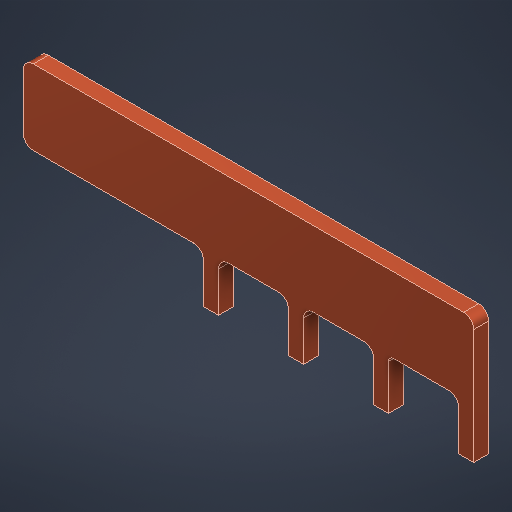
# Autodesk Inventor part: Bus_copper_GND
Saved by Autodesk Inventor 2026.2 (Build 302298000, 298)
## iProperties
Created: 2025-12-09
Part Number: Bus_copper_GND
Material: Медь
Document SubType Name: Modeling
Designer: EV-TECH
Density: 8.94 g/cm^3
Appearance: Медь — сатинированная
Author: EV-TECH
Autodesk Inventor part; units mm, degrees
ref_plane "YZ Plane" through (0, 0, 0) normal (1, 0, 0) x (0, 1, 0)
ref_plane "XZ Plane" through (0, 0, 0) normal (0, 1, 0) x (-1, 0, 0)
ref_plane "XY Plane" through (0, 0, 0) normal (0, 0, 1) x (1, 0, 0)
sketch "Эскиз1" plane through (0, 0, 0) normal (0, 1, 0) x (-1, 0, 0)
  line L0 (0, 0) -> (3, 0)
  line L1 (3, 0) -> (3, -3)
  line L2 (3, -3) -> (0, -3)
  line L3 (0, -3) -> (0, 0)
  line L4 (3, 0) -> (20, 0)
  line L5 (20, 0) -> (17, 0)
  line L6 (17, 0) -> (17, -3)
  line L7 (17, -3) -> (20, -3)
  line L8 (20, -3) -> (20, 0)
  line L9 (20, 0) -> (37, 0)
  line L10 (37, 0) -> (34, 0)
  line L11 (34, 0) -> (34, -3)
  line L12 (34, -3) -> (37, -3)
  line L13 (37, -3) -> (37, 0)
  line L14 (37, 0) -> (54, 0)
  line L15 (54, 0) -> (51, 0)
  line L16 (51, 0) -> (51, -3)
  line L17 (51, -3) -> (54, -3)
  line L18 (54, -3) -> (54, 0)
  point P0 (17, 0)
  point P1 (17, 0)
  dimension "d0" = 3
  dimension "d1" = 3
  dimension "d17" = 17
  dimension "d18" = 3
  dimension "d19" = 3
  dimension "d20" = 17
  dimension "d21" = 17
  dimension "d22" = 3
  dimension "d23" = 3
  dimension "d24" = 3
  dimension "d25" = 3
  constraints: 38 end point, 8 parallel, 7 horizontal, 4 perpendicular, 1 point on line
  measures "d0" distance of L1.end L2.end
  measures "d1" distance of L0.end L1.end
  measures "d17" distance of L0.end L4.end
  measures "d18" distance of L6.end L7.end
  measures "d19" distance of L7.end L4.end
  measures "d20" distance of L4.end L9.end
  measures "d21" distance of L9.end L14.end
  measures "d22" distance of L16.end L17.end
  measures "d23" distance of L17.end L14.end
  measures "d24" distance of L12.end L9.end
  measures "d25" distance of L11.end L12.end
extrude "Выдавливание1" add sketch "Эскиз1" along normal blind 10
sketch "Эскиз2" plane through (0, 10, 0) normal (0, 1, 0) x (1, 0, 0)
  line L0 (0, 0) -> (-90, 0)
  line L1 (-90, 0) -> (-90, 3)
  line L2 (-90, 3) -> (0, 3)
  line L3 (0, 3) -> (0, 0)
  dimension "d13" = 3
  dimension "d14" = 90
  constraints: 8 end point, 2 parallel, 1 horizontal, 1 perpendicular
  measures "d13" distance of L0.end L1.end
  measures "d14" distance of L1.end L2.end
extrude "Выдавливание2" add sketch "Эскиз2" along normal blind 15
fillet "Сопряжение1" radius 1 1 edges at (-17, 10, -1.5)
fillet "Сопряжение2" radius 2 7 edges at (-34, 10, -1.5) (-51, 10, -1.5) (-54, 10, -1.5) (-37, 10, -1.5) (-20, 10, -1.5) (-3, 10, -1.5) (0, 25, -1.5)
fillet "Сопряжение3" radius 2 2 edges at (-90, 25, -1.5) (-90, 10, -1.5)
